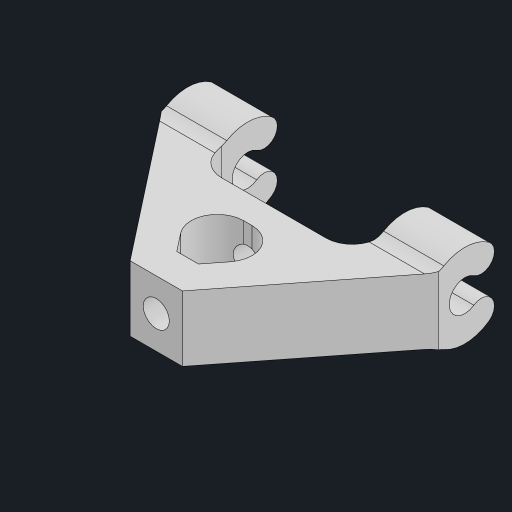
# Autodesk Inventor part: om_gear_base1
Saved by Autodesk Inventor 2023 (Build 270158000, 158)
## iProperties
Created: 2022-06-15
Part Number: om_gear_base1
Material: 一般
Document SubType Name: Modeling
Designer: legot
Density: 1 g/cm^3
Appearance: 既定
Author: legot
Autodesk Inventor part; units mm, degrees
ref_plane "YZ Plane" through (0, 0, 0) normal (1, 0, 0) x (0, 1, 0)
ref_plane "XZ Plane" through (0, 0, 0) normal (0, 1, 0) x (-1, 0, 0)
ref_plane "XY Plane" through (0, 0, 0) normal (0, 0, 1) x (1, 0, 0)
sketch "スケッチ1" plane through (0, 0, 0) normal (0, 1, 0) x (-1, 0, 0)
  line L0 (10.6147, -2) -> (-10.6147, -2)
  line L1 (-10.6147, -2) -> (-10.6147, 2)
  line L2 (10.6147, 2) -> (10.6147, -2)
  line L3 (10.6147, 2) -> (2, 13)
  line L4 (2, 13) -> (-2, 13)
  line L5 (-2, 13) -> (-10.6147, 2)
  line L6 (4.4337, 6) -> (0.8312, 10.6)
  line L7 (0.8312, 10.6) -> (-0.8312, 10.6)
  line L8 (-0.8312, 10.6) -> (-4.4337, 6)
  line L9 (6, 4) -> (-6, 4)
  line L10 (4.4337, 6) -> (-4.4337, 6)
  line L11 (6, 4) -> (6, -2)
  line L12 (-6, 4) -> (-6, -2)
  point P0 (0, 0)
  point P1 (10.6147, 0)
  point P2 (0, -2)
  point P3 (0, 13)
  dimension "d1" = 4
  dimension "d2" = 4
  dimension "d3" = 13
  dimension "d4" = 2.4
  dimension "d18" = 2
  dimension "d19" = 4
  dimension "d29" = 12
  constraints: 28 end point, 4 point on line, 3 horizontal, 3 midpoint, 3 parallel, 2 perpendicular, 2 vertical alignment, 1 equal length, 1 horizontal alignment, 2 other
  measures "d1" distance of L2.start L0.start
  measures "d2" distance of L3.end L4.end
  measures "d3" distance from line of point (0, 0) L4
  measures "d4" distance between parallel lines of L8 L5
  measures "d18" distance between parallel lines of L9 L10
  measures "d19" distance from line of L9 point (0, 0)
  measures "d29" distance between parallel lines of L12 L11
extrude "押し出し1" add sketch "スケッチ1" along normal mid plane 5 contours L0 L11 L9 L12 L1 L5 L4 L3 L2
sketch "スケッチ3" plane through (-2, 2.5, 13) normal (0, 0, 1) x (1, 0, 0)
  point P0 (2, -2.5)
  point P1 (2, -2.5)
  constraints: 1 coincident
hole "穴1" at (0, 0, 13) direction (0, 0, -1) diameter 2 end through all
sketch "スケッチ4" plane through (10.6147, -2.5, -2) normal (1, 0, 0) x (0, 0, -1)
  line L0 (0, 5) -> (0, 0) projected
  line L1 (-4, 0) -> (-4, 5) projected
  line L2 (0, 0) -> (-4, 0) projected
  circle A0 centre (-2, 2.5) radius 1.2
  line L3 (-4, 5) -> (0, 5) projected
  arc A1 (-4, 0) -> (-4, 5) centre (-2, 2.5) ccw
  circle A2 centre (-0.7377, 4.3028) radius 1.0008
  circle A3 centre (-0.7377, 0.6972) radius 1.0008
  line L4 (-0.7377, 4.3028) -> (-2, 2.5) construction
  line L5 (-2, 2.5) -> (-0.7377, 0.6972) construction
  line L6 (-0.7377, 1.698) -> (-0.7377, 3.302) construction
  line L7 (0, 2.2089) -> (-0.7377, 4.3028) construction
  point P0 (-1.3117, 3.483)
  point P1 (-1.3117, 1.517)
  point P2 (-0.0197, 0)
  point P3 (-0.0197, 5)
  point P4 (-0.1637, 5.1226)
  point P5 (-0.1637, -0.1226)
  dimension "d22" = 2.0016
  dimension "d20" = 2.4
  dimension "d21" = 110
  dimension "d23" = 1.604
  constraints: 10 end point, 3 point on circle, 3 point on line, 2 centre point, 2 coincident, 1 vertical alignment, 10 other
  measures "d20" diameter of A0
  measures "d21" angle of L5 L4
  measures "d23" distance of L6.start L6.end
extrude "押し出し3" add sketch "スケッチ4" against normal up to surface (4.6147 mm away)
extrude "押し出し4" cut sketch "スケッチ4" against normal up to surface (4.6147 mm away) contours A1 L0 A3 A2 | L0 A2 L3 | L3 A2 A1 | L2 A3 L0 | A1 A3 L2 | L0 A3 A0 A2 | A0 picked at (-0.0065, 4.9931) picked at (-0.0245, 5.014) picked at (-0.0065, 0.0069) picked at (-0.0245, -0.014)
mirror "ミラー1" about plane through (0, 0, 0) normal (1, 0, 0) of "押し出し3", "押し出し4"
fillet "フィレット2" radius 2 8 edges at (-6, 0, 4) (-4.4337, 0, 6) (6, 0, 4) (4.4337, 0, 6) (-8.3074, 2.5, 2) (8.3074, 2.5, 2) (8.3074, -2.5, 2) (-8.3074, -2.5, 2)
